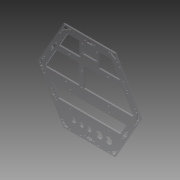
# Autodesk Inventor part: Top Plate
Saved by Autodesk Inventor 2015 (Build 190159000, 159)
## iProperties
Created: 2015-11-27
Part Number: Top Plate
Material: Polycarbonate, Clear
Document SubType Name: Modeling
Designer: James
Density: 1.2 g/cm^3
Appearance: Polycarbonate - Clear
Mass: 22.9754 g
Surface Area: 179.683 cm^2
Volume: 19.1462 cm^3
Author: James
Autodesk Inventor part; units mm, degrees
ref_plane "YZ Plane" through (0, 0, 0) normal (1, 0, 0) x (0, 1, 0)
ref_plane "XZ Plane" through (0, 0, 0) normal (0, 1, 0) x (-1, 0, 0)
ref_plane "XY Plane" through (0, 0, 0) normal (0, 0, 1) x (1, 0, 0)
sketch "Sketch1" plane through (0, 0, 0) normal (0, 1, 0) x (-1, 0, 0)
  line L0 (-150, 86.6025) -> (-200, 0)
  line L1 (-200, 0) -> (-150, -86.6025)
  line L2 (-150, -86.6025) -> (-50, -86.6025)
  line L3 (-50, -86.6025) -> (0, 0)
  line L4 (0, 0) -> (-50, 86.6025)
  line L5 (-50, 86.6025) -> (-150, 86.6025)
  line L6 (-100, 77.6025) -> (-94.5, 77.6025)
  line L7 (-94.5, 77.6025) -> (-94.5, 81.8025)
  line L8 (-105.5, 81.8025) -> (-105.5, 77.6025)
  line L9 (-105.5, 77.6025) -> (-100, 77.6025)
  arc A0 (-97.4544, 81.8025) -> (-102.5456, 81.8025) centre (-100, 80.9025) ccw
  line L10 (-105.5, 81.8025) -> (-102.5456, 81.8025)
  line L11 (-97.4544, 81.8025) -> (-94.5, 81.8025)
  line L12 (-145.5, 78.8083) -> (-140.7369, 81.5583)
  line L13 (-140.7369, 81.5583) -> (-142.8369, 85.1956)
  line L14 (-152.3631, 79.6956) -> (-150.2631, 76.0583)
  line L15 (-150.2631, 76.0583) -> (-145.5, 78.8083)
  arc A1 (-145.3955, 83.7184) -> (-149.8045, 81.1728) centre (-147.15, 81.6662) ccw
  line L16 (-152.3631, 79.6956) -> (-149.8045, 81.1728)
  line L17 (-145.3955, 83.7184) -> (-142.8369, 85.1956)
  line L18 (-167.2058, 38.8013) -> (-164.4558, 43.5644)
  line L19 (-164.4558, 43.5644) -> (-168.0931, 45.6644)
  line L20 (-173.5931, 36.1381) -> (-169.9558, 34.0381)
  line L21 (-169.9558, 34.0381) -> (-167.2058, 38.8013)
  arc A2 (-169.5703, 43.1058) -> (-172.1159, 38.6967) centre (-170.0637, 40.4513) ccw
  line L22 (-173.5931, 36.1381) -> (-172.1159, 38.6967)
  line L23 (-169.5703, 43.1058) -> (-168.0931, 45.6644)
  line L24 (-191, 0) -> (-191, 5.5)
  line L25 (-191, 5.5) -> (-195.2, 5.5)
  line L26 (-195.2, -5.5) -> (-191, -5.5)
  line L27 (-191, -5.5) -> (-191, 0)
  arc A3 (-195.2, 2.5456) -> (-195.2, -2.5456) centre (-194.3, 0) ccw
  line L28 (-195.2, -5.5) -> (-195.2, -2.5456)
  line L29 (-195.2, 2.5456) -> (-195.2, 5.5)
  line L30 (-167.2058, -38.8013) -> (-169.9558, -34.0381)
  line L31 (-169.9558, -34.0381) -> (-173.5931, -36.1381)
  line L32 (-168.0931, -45.6644) -> (-164.4558, -43.5644)
  line L33 (-164.4558, -43.5644) -> (-167.2058, -38.8013)
  arc A4 (-172.1159, -38.6967) -> (-169.5703, -43.1058) centre (-170.0637, -40.4513) ccw
  line L34 (-168.0931, -45.6644) -> (-169.5703, -43.1058)
  line L35 (-172.1159, -38.6967) -> (-173.5931, -36.1381)
  line L36 (-145.5, -78.8083) -> (-150.2631, -76.0583)
  line L37 (-150.2631, -76.0583) -> (-152.3631, -79.6956)
  line L38 (-142.8369, -85.1956) -> (-140.7369, -81.5583)
  line L39 (-140.7369, -81.5583) -> (-145.5, -78.8083)
  arc A5 (-149.8045, -81.1728) -> (-145.3955, -83.7184) centre (-147.15, -81.6662) ccw
  line L40 (-142.8369, -85.1956) -> (-145.3955, -83.7184)
  line L41 (-149.8045, -81.1728) -> (-152.3631, -79.6956)
  line L42 (-100, -77.6025) -> (-105.5, -77.6025)
  line L43 (-105.5, -77.6025) -> (-105.5, -81.8025)
  line L44 (-94.5, -81.8025) -> (-94.5, -77.6025)
  line L45 (-94.5, -77.6025) -> (-100, -77.6025)
  arc A6 (-102.5456, -81.8025) -> (-97.4544, -81.8025) centre (-100, -80.9025) ccw
  line L46 (-94.5, -81.8025) -> (-97.4544, -81.8025)
  line L47 (-102.5456, -81.8025) -> (-105.5, -81.8025)
  line L48 (-54.5, -78.8083) -> (-59.2631, -81.5583)
  line L49 (-59.2631, -81.5583) -> (-57.1631, -85.1956)
  line L50 (-47.6369, -79.6956) -> (-49.7369, -76.0583)
  line L51 (-49.7369, -76.0583) -> (-54.5, -78.8083)
  arc A7 (-54.6045, -83.7184) -> (-50.1955, -81.1728) centre (-52.85, -81.6662) ccw
  line L52 (-47.6369, -79.6956) -> (-50.1955, -81.1728)
  line L53 (-54.6045, -83.7184) -> (-57.1631, -85.1956)
  line L54 (-32.7942, -38.8013) -> (-35.5442, -43.5644)
  line L55 (-35.5442, -43.5644) -> (-31.9069, -45.6644)
  line L56 (-26.4069, -36.1381) -> (-30.0442, -34.0381)
  line L57 (-30.0442, -34.0381) -> (-32.7942, -38.8013)
  arc A8 (-30.4297, -43.1058) -> (-27.8841, -38.6967) centre (-29.9363, -40.4513) ccw
  line L58 (-26.4069, -36.1381) -> (-27.8841, -38.6967)
  line L59 (-30.4297, -43.1058) -> (-31.9069, -45.6644)
  line L60 (-9, 0) -> (-9, -5.5)
  line L61 (-9, -5.5) -> (-4.8, -5.5)
  line L62 (-4.8, 5.5) -> (-9, 5.5)
  line L63 (-9, 5.5) -> (-9, 0)
  arc A9 (-4.8, -2.5456) -> (-4.8, 2.5456) centre (-5.7, 0) ccw
  line L64 (-4.8, 5.5) -> (-4.8, 2.5456)
  line L65 (-4.8, -2.5456) -> (-4.8, -5.5)
  line L66 (-32.7942, 38.8013) -> (-30.0442, 34.0381)
  line L67 (-30.0442, 34.0381) -> (-26.4069, 36.1381)
  line L68 (-31.9069, 45.6644) -> (-35.5442, 43.5644)
  line L69 (-35.5442, 43.5644) -> (-32.7942, 38.8013)
  arc A10 (-27.8841, 38.6967) -> (-30.4297, 43.1058) centre (-29.9363, 40.4513) ccw
  line L70 (-31.9069, 45.6644) -> (-30.4297, 43.1058)
  line L71 (-27.8841, 38.6967) -> (-26.4069, 36.1381)
  line L72 (-54.5, 78.8083) -> (-49.7369, 76.0583)
  line L73 (-49.7369, 76.0583) -> (-47.6369, 79.6956)
  line L74 (-57.1631, 85.1956) -> (-59.2631, 81.5583)
  line L75 (-59.2631, 81.5583) -> (-54.5, 78.8083)
  arc A11 (-50.1955, 81.1728) -> (-54.6045, 83.7184) centre (-52.85, 81.6662) ccw
  line L76 (-57.1631, 85.1956) -> (-54.6045, 83.7184)
  line L77 (-50.1955, 81.1728) -> (-47.6369, 79.6956)
  circle A12 centre (-173.4244, 32.2302) radius 1.6
  circle A13 centre (-164.6244, 47.4723) radius 1.6
  circle A14 centre (-164.6244, -47.4723) radius 1.6
  circle A15 centre (-173.4244, -32.2302) radius 1.6
  circle A16 centre (-91.2, -79.7025) radius 1.6
  circle A17 centre (-108.8, -79.7025) radius 1.6
  circle A18 centre (-26.5756, -32.2302) radius 1.6
  circle A19 centre (-35.3756, -47.4723) radius 1.6
  circle A20 centre (-35.3756, 47.4723) radius 1.6
  circle A21 centre (-26.5756, 32.2302) radius 1.6
  circle A22 centre (-108.8, 79.7025) radius 1.6
  circle A23 centre (-91.2, 79.7025) radius 1.6
  circle A24 centre (-191, -8.8) radius 1.6
  circle A25 centre (-191, 8.8) radius 1.6
  circle A26 centre (-137.879, -83.2083) radius 1.6
  circle A27 centre (-153.121, -74.4083) radius 1.6
  circle A28 centre (-46.879, -74.4083) radius 1.6
  circle A29 centre (-62.121, -83.2083) radius 1.6
  circle A30 centre (-9, 8.8) radius 1.6
  circle A31 centre (-9, -8.8) radius 1.6
  circle A32 centre (-62.121, 83.2083) radius 1.6
  circle A33 centre (-46.879, 74.4083) radius 1.6
  circle A34 centre (-153.121, 74.4083) radius 1.6
  circle A35 centre (-137.879, 83.2083) radius 1.6
  circle A36 centre (-135.5474, 41.0731) radius 1.6079
  circle A37 centre (-84.7865, 25.8384) radius 1.6079
  circle A38 centre (-60.6651, 41.0731) radius 1.6079
  circle A39 centre (-84.7865, -2.0705) radius 1.6079
  circle A40 centre (-54.3385, -7.1487) radius 1.6079
  circle A41 centre (-136.817, -7.1487) radius 1.6079
  circle A42 centre (-137.5, -48.1487) radius 1.25
  circle A43 centre (-137.5, -17.1487) radius 1.25
  circle A44 centre (-62.5, -17.1487) radius 1.25
  circle A45 centre (-62.5, -48.1487) radius 1.25
  line L78 (-60.6651, 36.0731) -> (-35.8268, 36.0731)
  line L79 (-35.8268, 36.0731) -> (-79.7865, 36.0731)
  line L80 (-89.7865, -2.1487) -> (-183.7594, -2.1487)
  line L81 (-172.2124, -22.1487) -> (-27.7876, -22.1487)
  line L82 (-79.7865, -2.1487) -> (-16.2406, -2.1487)
  line L83 (-89.7865, 25.8384) -> (-89.7865, -2.1487)
  line L84 (-89.7865, -2.1487) -> (-89.7865, 36.0731)
  line L85 (-79.7865, 25.8384) -> (-79.7865, -2.1487)
  line L86 (-79.7865, -2.1487) -> (-79.7865, 36.0731)
  line L87 (-89.7865, 36.0731) -> (-164.1732, 36.0731)
  line L88 (-183.7594, -2.1487) -> (-185, 0)
  line L89 (-185, 0) -> (-164.1732, 36.0731)
  line L90 (-35.8268, 36.0731) -> (-15, 0)
  line L91 (-15, 0) -> (-16.2406, -2.1487)
  line L92 (-137.5, -43.1487) -> (-39.9119, -43.1487)
  line L93 (-137.5, -43.1487) -> (-160.0881, -43.1487)
  line L94 (-172.2124, -22.1487) -> (-160.0881, -43.1487)
  line L95 (-39.9119, -43.1487) -> (-27.7876, -22.1487)
  circle A46 centre (-137.5, -64.9519) radius 6.5
  circle A47 centre (-119.5, -64.9519) radius 6.5
  circle A48 centre (-99.9229, -64.9519) radius 4.5
  circle A49 centre (-99.9229, -64.9519) radius 4.5
  circle A50 centre (-84.9229, -64.9519) radius 4.5
  circle A51 centre (-69.9229, -64.9519) radius 4.5
  circle A52 centre (-114, 56.1025) radius 1.25
  circle A53 centre (-114, 71.1025) radius 1.25
  circle A54 centre (-86, 71.1025) radius 1.25
  circle A55 centre (-86, 56.1025) radius 1.25
  line L96 (-87.8, 57.6025) -> (-87.8, 54.6025)
  line L97 (-87.8, 54.6025) -> (-112.2, 54.6025)
  line L98 (-112.2, 54.6025) -> (-112.2, 57.6025)
  line L99 (-112.2, 57.6025) -> (-87.8, 57.6025)
  line L100 (-135.5474, 46.0731) -> (-119, 46.0731)
  line L101 (-119, 56.1025) -> (-119, 46.0731)
  line L102 (-158.3997, 46.0731) -> (-135.5474, 46.0731)
  line L103 (-142.5, 73.6122) -> (-158.3997, 46.0731)
  line L104 (-142.5, 73.6122) -> (-119, 73.6122)
  line L105 (-119, 73.6122) -> (-119, 56.1025)
  line L106 (-64.4526, 46.0731) -> (-81, 46.0731)
  line L107 (-81, 56.1025) -> (-81, 46.0731)
  line L108 (-41.6003, 46.0731) -> (-64.4526, 46.0731)
  line L109 (-57.5, 73.6122) -> (-41.6003, 46.0731)
  line L110 (-57.5, 73.6122) -> (-81, 73.6122)
  line L111 (-81, 73.6122) -> (-81, 56.1025)
  circle A56 centre (-117.305, -83.1025) radius 1.6
  circle A57 centre (-82.695, -83.1025) radius 1.6
  circle A58 centre (-187.7076, -13.5757) radius 1.6
  circle A59 centre (-187.7076, 13.5757) radius 1.6
  circle A60 centre (-12.2924, -13.5757) radius 1.6
  circle A61 centre (-12.2924, 13.5757) radius 1.6
  circle A62 centre (-157.387, 68.1524) radius 1.6
  circle A63 centre (-42.613, 68.1524) radius 1.6
  constraints: 224 end point, 64 centre point, 24 point on circle, 3 point on line
extrude "Extrusion3" add sketch "Sketch1" along normal blind 3
body "Solid3"
